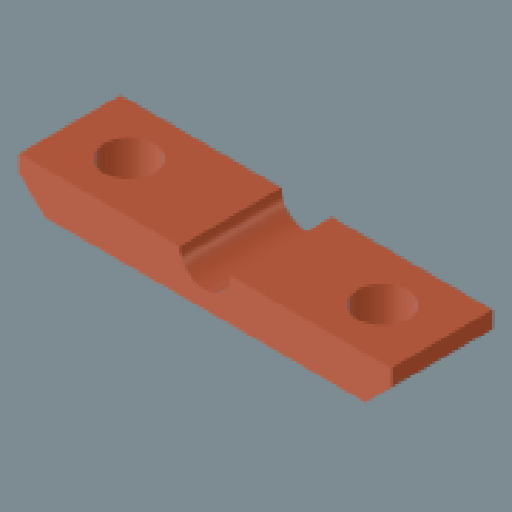
# Autodesk Inventor part: Idler Thermistor Clamp
Saved by Autodesk Inventor 2023.2 (Build 272271000, 271)
## iProperties
Created: 2023-02-14
Part Number: Idler Thermistor Clamp
Material: ABS Plastic
Document SubType Name: Modeling
Designer: remop
Density: 1.06 g/cm^3
Appearance: Smooth - Light Orange
Author: remop
Autodesk Inventor part; units mm, degrees
ref_plane "YZ Plane" through (0, 0, 0) normal (1, 0, 0) x (0, 1, 0)
ref_plane "XZ Plane" through (0, 0, 0) normal (0, 1, 0) x (-1, 0, 0)
ref_plane "XY Plane" through (0, 0, 0) normal (0, 0, 1) x (1, 0, 0)
sketch "Sketch1" plane through (0, 0, 0) normal (0, 0, 1) x (1, 0, 0)
  circle A0 centre (0, 0) radius 1.5
  line L0 (-10.5, -2.5) -> (10.5, -2.5)
  line L1 (-1.5, 0) -> (-1.5, 1.5)
  line L2 (-1.5, 1.5) -> (-10.5, 1.5)
  line L3 (-10.5, 1.5) -> (-10.5, -2.5)
  line L4 (1.5, 0) -> (1.5, 1.5)
  line L5 (1.5, 1.5) -> (10.5, 1.5)
  line L6 (10.5, 1.5) -> (10.5, -2.5)
  dimension "d0" = 3
  dimension "d1" = 21
  dimension "d17" = 2.5
  constraints: 14 end point, 3 perpendicular, 3 tangent, 2 point on circle, 2 point on line, 1 centre point, 1 coincident, 1 collinear, 1 horizontal, 1 parallel, 1 vertical
  measures "d0" diameter of A0
  measures "d1" distance of L0.start L0.end
  measures "d17" distance from line of L0 point (0, 0)
extrude "Extrusion1" add sketch "Sketch1" along normal blind 6 contours L4 L5 L6 L0 L3 L2 L1 A0
chamfer "Chamfer1" distance 1 angle 45 2 edges at (10.5, -2.5, 3) (-10.5, -2.5, 3)
sketch "Sketch3" plane through (-10.5, 1.5, 0) normal (0, 1, 0) x (1, 0, 0)
  line L0 (9, 0) -> (0, 0) projected
  line L1 (0, 0) -> (0, -6) projected
  line L2 (9, -6) -> (0, -6) projected
  line L3 (9, 0) -> (9, -6) projected
  line L4 (21, 0) -> (12, 0) projected
  line L5 (12, 0) -> (12, -6) projected
  line L6 (21, -6) -> (12, -6) projected
  line L7 (21, 0) -> (21, -6) projected
  point P0 (10.5, 0)
  point P1 (3, -3)
  point P2 (18, -3)
  point P3 (0, -3)
  point P4 (21, -3)
  dimension "d18" = 7.5
  dimension "d19" = 7.5
  constraints: 2 horizontal alignment, 2 midpoint
  measures "d18" horizontal distance of point (10.5, 0) point (3, -3)
  measures "d19" horizontal distance of point (18, -3) point (10.5, 0)
hole "Hole2" at (-7.5, 1.5, 3) at (7.5, 1.5, 3) direction (0, -1, 0) diameter 3 end through all
equation "\"d19\" = d18"
body "Solid1"
